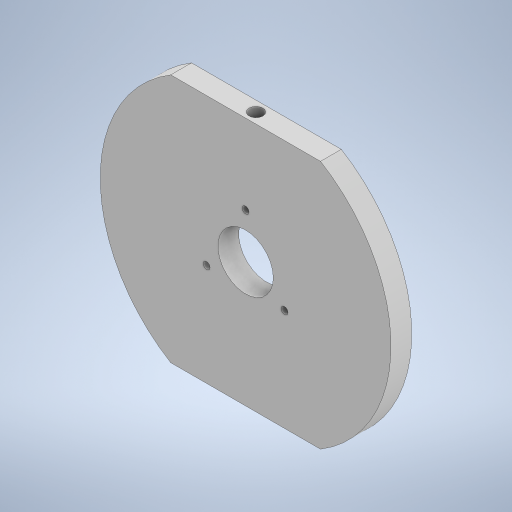
# Autodesk Inventor part: Tapa cvt
Saved by Autodesk Inventor 2023 (Build 270158000, 158)
## iProperties
Created: 2023-08-22
Part Number: Tapa cvt
Material: Genérico
Document SubType Name: Modeling
Designer: jpons
Density: 1 g/cm^3
Appearance: Valor por defecto
Author: jpons
Autodesk Inventor part; units mm, degrees
ref_plane "YZ Plane" through (0, 0, 0) normal (1, 0, 0) x (0, 1, 0)
ref_plane "XZ Plane" through (0, 0, 0) normal (0, 1, 0) x (-1, 0, 0)
sketch "Boceto1" plane through (0, 0, 0) normal (0, 0, 1) x (1, 0, 0)
  circle A0 centre (0, 0) radius 20
  line L0 (0, 0) -> (0, 37.5) construction
  line L1 (0, 0) -> (-32.476, -18.75) construction
  line L2 (0, 0) -> (32.476, -18.75) construction
  circle A1 centre (0, 0) radius 27.5 construction
  circle A2 centre (0, 32.5) radius 2.5
  circle A3 centre (-28.1458, -16.25) radius 2.5
  circle A4 centre (28.1458, -16.25) radius 2.5
  line L3 (0, 37.5) -> (0, 105) construction
  line L4 (-54.0833, 90) -> (54.0833, 90)
  line L5 (54.0833, -90) -> (-54.0833, -90)
  arc A5 (-54.0833, 90) -> (-54.0833, -90) centre (0, 0) ccw
  arc A6 (54.0833, -90) -> (54.0833, 90) centre (0, 0) ccw
  point P0 (0, 27.5)
  dimension "d2" = 55
  dimension "d1" = 40
  dimension "d3" = 10
  dimension "d4" = 120
  dimension "d5" = 120
  dimension "d6" = 120
  dimension "d7" = 5
  dimension "d8" = 5
  dimension "d11" = 360
  dimension "d13" = 90
  dimension "d16" = 360
  dimension "d18" = 105
  constraints: 12 end point, 6 centre point, 4 coincident, 4 point on circle, 3 point on line, 2 equal length, 1 horizontal, 1 perpendicular, 1 vertical, 1 vertical alignment, 16 other
  measures "d1" diameter of A0
  measures "d3" distance of L0.end point (0, 27.5)
  measures "d4" angle of L1 L0
  measures "d5" angle of L2 L1
  measures "d6" angle of L0 L2
  measures "d7" diameter of A2
  measures "d8" distance of point (0, 27.5) point (0, 32.5)
  measures "d13" distance from line of point (0, 0) L4
  measures "d18" radius of A6
extrude "Extrusión1" add sketch "Boceto1" along normal blind 15
sketch "Boceto2" plane through (-54.0833, 90, 0) normal (0, 1, 0) x (1, 0, 0)
  line L0 (54.0833, 0) -> (54.0833, -15) construction
  line L1 (108.1665, -15) -> (0, -15) construction
  line L2 (0, 0) -> (0, -15) construction
  line L3 (0, -7.5) -> (108.1665, -7.5) construction
  line L4 (108.1665, 0) -> (108.1665, -15) construction
  circle A0 centre (54.0833, -7.5) radius 5
  dimension "d21" = 10
  constraints: 4 end point, 4 midpoint, 1 centre point
  measures "d21" diameter of A0
extrude "Extrusión2" cut sketch "Boceto2" against normal blind 20
ref_plane "Plano de trabajo1" through (-105, 0, 15) normal (0, 1, 0) x (1, 0, 0)
mirror "Simetría1" about plane through (-105, 0, 15) normal (0, 1, 0) of "Extrusión2"
